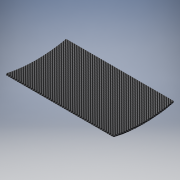
# Autodesk Inventor part: element_1
Saved by Autodesk Inventor 2018.1 (Build 221171000, 171)
## iProperties
Created: 2017-10-18
Part Number: element_1
Material: CFRP
Document SubType Name: Modeling
Designer: kuwano
Density: 1.43 g/cm^3
Appearance: カーボンファイバー
Mass: 74.8595 g
Surface Area: 365.403 cm^2
Volume: 52.3493 cm^3
Author: kuwano
Autodesk Inventor part; units mm, degrees
ref_plane "YZ Plane" through (0, 0, 0) normal (1, 0, 0) x (0, 1, 0)
ref_plane "XZ Plane" through (0, 0, 0) normal (0, 1, 0) x (-1, 0, 0)
ref_plane "XY Plane" through (0, 0, 0) normal (0, 0, 1) x (1, 0, 0)
sketch "スケッチ1" plane through (0, 0, 0) normal (1, 0, 0) x (0, 1, 0)
  arc A0 (8.4759, 50) -> (8.4759, -50) centre (234.0113, 0) ccw
  arc A1 (5.547, 50.6493) -> (5.547, -50.6493) centre (234.0113, 0) ccw
  line L0 (8.4759, 50) -> (5.547, 50.6493)
  line L1 (8.4759, -50) -> (5.547, -50.6493)
  line L2 (0, -70.909) -> (0, 70.909) projected
  point P0 (0, 0)
  point P1 (0, 0)
  dimension "d0" = 3
  dimension "d1" = 100
  dimension "d2" = 25
  constraints: 5 point on circle, 4 end point, 4 line through centre, 2 centre point, 1 coincident, 1 concentric, 1 tangent
  measures "d0" distance of L0.start L0.end
  measures "d1" distance of L1.start L0.start
  measures "d2" angle of L1 L0
extrude "押し出し1" add sketch "スケッチ1" along normal blind 180
sketch "スケッチ2" plane through (0, 0, 0) normal (-1, 0, 0) x (0, 0, 1)
  line L0 (-50.6493, 5.547) -> (-50, 8.4759) projected
  line L1 (-50.5452, 6.0168) -> (-35.9007, 2.7702)
  arc A0 (-50.6493, 5.547) -> (50.6493, 5.547) centre (0, 234.0113) ccw projected
  line L2 (-50, 8.4759) -> (-50.6493, 5.547) projected
  point P0 (0, 0)
  dimension "d5" = 15
  constraints: 2 end point, 1 perpendicular, 1 point on circle, 1 point on line
  measures "d5" distance of L1.start L1.end
extrude "押し出し2" cut sketch "スケッチ2" against normal through all
mirror "ミラー1" about plane through (0, 0, 0) normal (0, 0, 1) of "押し出し2"
